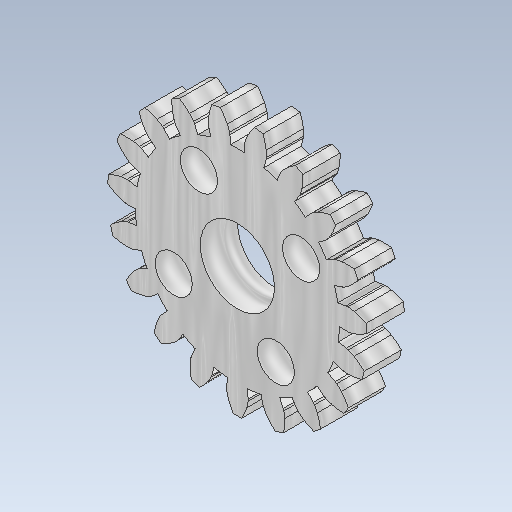
# Autodesk Inventor part: m1歯数19ギアネジ切3td5.98
Saved by Autodesk Inventor 2020.2 (Build 242310000, 310)
## iProperties
Created: 2020-02-29
Part Number: m1歯数19ギアネジ切3td5.98
Material: アルミニウム 7075
Document SubType Name: Modeling
Designer: aoyam
Density: 2.81 g/cm^3
Appearance: サテン - ブラシ仕上げ 重厚
Author: aoyam
Autodesk Inventor part; units mm, degrees
ref_plane "YZ Plane" through (0, 0, 0) normal (1, 0, 0) x (0, 1, 0)
ref_plane "XZ Plane" through (0, 0, 0) normal (0, 1, 0) x (-1, 0, 0)
ref_plane "XY Plane" through (0, 0, 0) normal (0, 0, 1) x (1, 0, 0)
sketch "スケッチ1" plane through (0, 0, 0) normal (0, 0, 1) x (1, 0, 0)
  arc A0 (2.202, 9.4851) -> (2.1723, 9.3327) centre (3.0999, 9.2311) ccw
  arc A1 (2.3854, 9.9626) -> (2.202, 9.4851) centre (4.6851, 8.8056) ccw
  arc A2 (2.953, 10.829) -> (2.3854, 9.9626) centre (6.3936, 7.9557) ccw
  arc A3 (0.9673, 9.3327) -> (0.9376, 9.4851) centre (0.0398, 9.2311) ccw
  arc A4 (0.9376, 9.4851) -> (0.7543, 9.9626) centre (-1.5454, 8.8056) ccw
  arc A5 (0.7543, 9.9626) -> (0.1867, 10.829) centre (-3.2539, 7.9557) ccw
  arc A6 (2.1266, 8.6594) -> (1.013, 8.6594) centre (1.5698, 0.4558) ccw
  arc A7 (0.1867, 10.829) -> (-0.4901, 10.716) centre (1.5698, 0.4558) ccw
  line L0 (2.1266, 8.6594) -> (2.1723, 9.3327)
  line L1 (1.013, 8.6594) -> (0.9673, 9.3327)
  line L2 (-1.6205, 8.0341) -> (-1.8823, 8.6561)
  arc A8 (-1.8823, 8.6561) -> (-1.9599, 8.7906) centre (-2.7267, 8.2588) ccw
  arc A9 (-1.9599, 8.7906) -> (-2.2884, 9.1827) centre (-4.0878, 7.3416) ccw
  arc A10 (-2.2884, 9.1827) -> (-3.1065, 9.8178) centre (-5.4278, 5.983) ccw
  arc A11 (-3.1065, 9.8178) -> (-3.71, 9.4912) centre (1.5698, 0.4558) ccw
  arc A12 (-0.764, 9.2012) -> (-0.7426, 9.0473) centre (0.1677, 9.2524) ccw
  arc A13 (-0.5672, 8.3957) -> (-1.6205, 8.0341) centre (1.5698, 0.4558) ccw
  line L3 (-0.5672, 8.3957) -> (-0.7426, 9.0473)
  arc A14 (-0.7457, 9.7123) -> (-0.764, 9.2012) centre (1.8051, 9.3647) ccw
  arc A15 (-0.4901, 10.716) -> (-0.7457, 9.7123) centre (3.697, 9.1156) ccw
  line L4 (-3.9083, 6.5876) -> (-4.3579, 7.0908)
  arc A16 (-4.3579, 7.0908) -> (-4.475, 7.1929) centre (-5.0275, 6.4409) ccw
  arc A17 (-4.475, 7.1929) -> (-4.9129, 7.4571) centre (-6.0171, 5.1315) ccw
  arc A18 (-4.9129, 7.4571) -> (-5.893, 7.7921) centre (-6.8433, 3.4114) ccw
  arc A19 (-5.893, 7.7921) -> (-6.3577, 7.2873) centre (1.5698, 0.4558) ccw
  arc A20 (-3.4772, 7.9695) -> (-3.407, 7.8309) centre (-2.6126, 8.3205) ccw
  arc A21 (-3.0295, 7.2716) -> (-3.9083, 6.5876) centre (1.5698, 0.4558) ccw
  line L5 (-3.0295, 7.2716) -> (-3.407, 7.8309)
  arc A22 (-3.6258, 8.4589) -> (-3.4772, 7.9695) centre (-1.1003, 8.9584) ccw
  arc A23 (-3.71, 9.4912) -> (-3.6258, 8.4589) centre (0.7699, 9.337) ccw
  line L6 (-5.6025, 4.4766) -> (-6.1911, 4.8066)
  arc A24 (-6.1911, 4.8066) -> (-6.335, 4.8651) centre (-6.6134, 3.9745) ccw
  arc A25 (-6.335, 4.8651) -> (-6.835, 4.9728) centre (-7.1242, 2.4147) ccw
  arc A26 (-6.835, 4.9728) -> (-7.8708, 4.9714) centre (-7.3472, 0.5195) ccw
  arc A27 (-7.8708, 4.9714) -> (-8.1464, 4.3431) centre (1.5698, 0.4558) ccw
  arc A28 (-5.6434, 5.9236) -> (-5.5321, 5.8154) centre (-4.9397, 6.5363) ccw
  arc A29 (-4.9934, 5.4089) -> (-5.6025, 4.4766) centre (1.5698, 0.4558) ccw
  line L7 (-4.9934, 5.4089) -> (-5.5321, 5.8154)
  arc A30 (-5.9429, 6.3382) -> (-5.6434, 5.9236) centre (-3.7165, 7.6307) ccw
  arc A31 (-6.3577, 7.2873) -> (-5.9429, 6.3382) centre (-2.0705, 8.5961) ccw
  line L8 (-6.5194, 1.9299) -> (-7.1833, 2.0508)
  arc A32 (-7.1833, 2.0508) -> (-7.3384, 2.0595) centre (-7.3126, 1.1267) ccw
  arc A33 (-7.3384, 2.0595) -> (-7.8463, 1.999) centre (-7.2892, -0.5144) ccw
  arc A34 (-7.8463, 1.999) -> (-8.8255, 1.6614) centre (-6.8847, -2.3793) ccw
  arc A35 (-8.8255, 1.6614) -> (-8.8821, 0.9776) centre (1.5698, 0.4558) ccw
  arc A36 (-7.028, 3.2852) -> (-6.8875, 3.219) centre (-6.5613, 4.0932) ccw
  arc A37 (-6.2461, 3.0094) -> (-6.5194, 1.9299) centre (1.5698, 0.4558) ccw
  line L9 (-6.2461, 3.0094) -> (-6.8875, 3.219)
  arc A38 (-7.4459, 3.5801) -> (-7.028, 3.2852) centre (-5.7597, 5.5255) ccw
  arc A39 (-8.1464, 4.3431) -> (-7.4459, 3.5801) centre (-4.5164, 6.973) ccw
  line L10 (-6.5598, -0.7766) -> (-7.227, -0.8777)
  arc A40 (-7.227, -0.8777) -> (-7.3765, -0.9199) centre (-7.0491, -1.7937) ccw
  arc A41 (-7.3765, -0.9199) -> (-7.8372, -1.1421) centre (-6.4942, -3.3384) ccw
  arc A42 (-7.8372, -1.1421) -> (-8.6537, -1.7793) centre (-5.5061, -4.9709) ccw
  arc A43 (-8.6537, -1.7793) -> (-8.4853, -2.4444) centre (1.5698, 0.4558) ccw
  arc A44 (-7.4809, 0.3402) -> (-7.3265, 0.3232) centre (-7.3019, 1.2559) ccw
  arc A45 (-6.6517, 0.3332) -> (-6.5598, -0.7766) centre (1.5698, 0.4558) ccw
  line L11 (-6.6517, 0.3332) -> (-7.3265, 0.3232)
  arc A46 (-7.9719, 0.4835) -> (-7.4809, 0.3402) centre (-7.0087, 2.8709) ccw
  arc A47 (-8.8821, 0.9776) -> (-7.9719, 0.4835) centre (-6.3028, 4.6437) ccw
  line L12 (-5.7192, -3.3495) -> (-6.3174, -3.6618)
  arc A48 (-6.3174, -3.6618) -> (-6.445, -3.7502) centre (-5.8517, -4.4704) ccw
  arc A49 (-6.445, -3.7502) -> (-6.8087, -4.1099) centre (-4.8253, -5.7512) ccw
  arc A50 (-6.8087, -4.1099) -> (-7.374, -4.9778) centre (-3.3607, -6.9744) ccw
  arc A51 (-7.374, -4.9778) -> (-6.9988, -5.5522) centre (1.5698, 0.4558) ccw
  arc A52 (-6.953, -2.5923) -> (-6.8014, -2.5583) centre (-7.081, -1.6681) ccw
  arc A53 (-6.1665, -2.3297) -> (-5.7192, -3.3495) centre (1.5698, 0.4558) ccw
  line L13 (-6.1665, -2.3297) -> (-6.8014, -2.5583)
  arc A54 (-7.4639, -2.6162) -> (-6.953, -2.5923) centre (-7.3281, -0.0455) ccw
  arc A55 (-8.4853, -2.4444) -> (-7.4639, -2.6162) centre (-7.236, 1.8605) ccw
  line L14 (-4.0886, -5.5101) -> (-4.553, -5.9997)
  arc A56 (-4.553, -5.9997) -> (-4.6451, -6.1248) centre (-3.8501, -6.6133) ccw
  arc A57 (-4.6451, -6.1248) -> (-4.8722, -6.5831) centre (-2.4634, -7.4914) ccw
  arc A58 (-4.8722, -6.5831) -> (-5.1252, -7.5874) centre (-0.681, -8.1727) ccw
  arc A59 (-5.1252, -7.5874) -> (-4.5837, -8.0089) centre (1.5698, 0.4558) ccw
  arc A60 (-5.5015, -5.1945) -> (-5.3692, -5.1131) centre (-5.9227, -4.3619) ccw
  arc A61 (-4.8429, -4.6907) -> (-4.0886, -5.5101) centre (1.5698, 0.4558) ccw
  line L15 (-4.8429, -4.6907) -> (-5.3692, -5.1131)
  arc A62 (-5.9769, -5.383) -> (-5.5015, -5.1945) centre (-6.6832, -2.9075) ccw
  arc A63 (-6.9988, -5.5522) -> (-5.9769, -5.383) centre (-7.2151, -1.0748) ccw
  line L16 (-1.845, -7.0241) -> (-2.1252, -7.638)
  arc A64 (-2.1252, -7.638) -> (-2.1717, -7.7862) centre (-1.2611, -7.9901) ccw
  arc A65 (-2.1717, -7.7862) -> (-2.2377, -8.2934) centre (0.3356, -8.3704) ccw
  arc A66 (-2.2377, -8.2934) -> (-2.1508, -9.3255) centre (2.2426, -8.4361) ccw
  arc A67 (-2.1508, -9.3255) -> (-1.5018, -9.5483) centre (1.5698, 0.4558) ccw
  arc A68 (-3.2837, -7.1844) -> (-3.185, -7.0645) centre (-3.9524, -6.5337) ccw
  arc A69 (-2.8243, -6.4941) -> (-1.845, -7.0241) centre (1.5698, 0.4558) ccw
  line L17 (-2.8243, -6.4941) -> (-3.185, -7.0645)
  arc A70 (-3.6722, -7.5171) -> (-3.2837, -7.1844) centre (-5.144, -5.405) ccw
  arc A71 (-4.5837, -8.0089) -> (-3.6722, -7.5171) centre (-6.2421, -3.8444) ccw
  line L18 (0.7688, -7.7276) -> (0.703, -8.3992)
  arc A72 (0.703, -8.3992) -> (0.7072, -8.5545) centre (1.6347, -8.4517) ccw
  arc A73 (0.7072, -8.5545) -> (0.8095, -9.0556) centre (3.2683, -8.2929) ccw
  arc A74 (0.8095, -9.0556) -> (1.2268, -10.0036) centre (5.0934, -7.7358) ccw
  arc A75 (1.2268, -10.0036) -> (1.9129, -10.0036) centre (1.5698, 0.4558) ccw
  arc A76 (-0.5399, -8.3464) -> (-0.4855, -8.2009) centre (-1.3837, -7.948) ccw
  arc A77 (-0.3296, -7.5443) -> (0.7688, -7.7276) centre (1.5698, 0.4558) ccw
  line L19 (-0.3296, -7.5443) -> (-0.4855, -8.2009)
  arc A78 (-0.7994, -8.7872) -> (-0.5399, -8.3464) centre (-2.8773, -7.2674) ccw
  arc A79 (-1.5018, -9.5483) -> (-0.7994, -8.7872) centre (-4.4226, -6.1479) ccw
  line L20 (3.4693, -7.5443) -> (3.6252, -8.2009)
  arc A80 (3.6252, -8.2009) -> (3.6796, -8.3464) centre (4.5234, -7.948) ccw
  arc A81 (3.6796, -8.3464) -> (3.939, -8.7872) centre (6.0169, -7.2674) ccw
  arc A82 (3.939, -8.7872) -> (4.6415, -9.5483) centre (7.5622, -6.1479) ccw
  arc A83 (4.6415, -9.5483) -> (5.2905, -9.3255) centre (1.5698, 0.4558) ccw
  arc A84 (2.4324, -8.5545) -> (2.4366, -8.3992) centre (1.505, -8.4517) ccw
  arc A85 (2.3709, -7.7276) -> (3.4693, -7.5443) centre (1.5698, 0.4558) ccw
  line L21 (2.3709, -7.7276) -> (2.4366, -8.3992)
  arc A86 (2.3302, -9.0556) -> (2.4324, -8.5545) centre (-0.1286, -8.2929) ccw
  arc A87 (1.9129, -10.0036) -> (2.3302, -9.0556) centre (-1.9537, -7.7358) ccw
  line L22 (5.964, -6.4941) -> (6.3247, -7.0645)
  arc A88 (6.3247, -7.0645) -> (6.4233, -7.1844) centre (7.0921, -6.5337) ccw
  arc A89 (6.4233, -7.1844) -> (6.8118, -7.5171) centre (8.2837, -5.405) ccw
  arc A90 (6.8118, -7.5171) -> (7.7234, -8.0089) centre (9.3818, -3.8444) ccw
  arc A91 (7.7234, -8.0089) -> (8.2649, -7.5874) centre (1.5698, 0.4558) ccw
  arc A92 (5.3113, -7.7862) -> (5.2649, -7.638) centre (4.4008, -7.9901) ccw
  arc A93 (4.9846, -7.0241) -> (5.964, -6.4941) centre (1.5698, 0.4558) ccw
  line L23 (4.9846, -7.0241) -> (5.2649, -7.638)
  arc A94 (5.3773, -8.2934) -> (5.3113, -7.7862) centre (2.8041, -8.3704) ccw
  arc A95 (5.2905, -9.3255) -> (5.3773, -8.2934) centre (0.897, -8.4361) ccw
  line L24 (7.9826, -4.6907) -> (8.5089, -5.1131)
  arc A96 (8.5089, -5.1131) -> (8.6411, -5.1945) centre (9.0623, -4.3619) ccw
  arc A97 (8.6411, -5.1945) -> (9.1166, -5.383) centre (9.8229, -2.9075) ccw
  arc A98 (9.1166, -5.383) -> (10.1384, -5.5522) centre (10.3547, -1.0748) ccw
  arc A99 (10.1384, -5.5522) -> (10.5137, -4.9778) centre (1.5698, 0.4558) ccw
  arc A100 (7.7848, -6.1248) -> (7.6927, -5.9997) centre (6.9898, -6.6133) ccw
  arc A101 (7.2283, -5.5101) -> (7.9826, -4.6907) centre (1.5698, 0.4558) ccw
  line L25 (7.2283, -5.5101) -> (7.6927, -5.9997)
  arc A102 (8.0119, -6.5831) -> (7.7848, -6.1248) centre (5.6031, -7.4914) ccw
  arc A103 (8.2649, -7.5874) -> (8.0119, -6.5831) centre (3.8207, -8.1727) ccw
  line L26 (9.3062, -2.3297) -> (9.9411, -2.5583)
  arc A104 (9.9411, -2.5583) -> (10.0926, -2.5923) centre (10.2207, -1.6681) ccw
  arc A105 (10.0926, -2.5923) -> (10.6035, -2.6162) centre (10.4678, -0.0455) ccw
  arc A106 (10.6035, -2.6162) -> (11.6249, -2.4444) centre (10.3757, 1.8605) ccw
  arc A107 (11.6249, -2.4444) -> (11.7934, -1.7793) centre (1.5698, 0.4558) ccw
  arc A108 (9.5847, -3.7502) -> (9.457, -3.6618) centre (8.9914, -4.4704) ccw
  arc A109 (8.8588, -3.3495) -> (9.3062, -2.3297) centre (1.5698, 0.4558) ccw
  line L27 (8.8588, -3.3495) -> (9.457, -3.6618)
  arc A110 (9.9483, -4.1099) -> (9.5847, -3.7502) centre (7.965, -5.7512) ccw
  arc A111 (10.5137, -4.9778) -> (9.9483, -4.1099) centre (6.5004, -6.9744) ccw
  line L28 (9.7914, 0.3332) -> (10.4662, 0.3232)
  arc A112 (10.4662, 0.3232) -> (10.6206, 0.3402) centre (10.4415, 1.2559) ccw
  arc A113 (10.6206, 0.3402) -> (11.1115, 0.4835) centre (10.1484, 2.8709) ccw
  arc A114 (11.1115, 0.4835) -> (12.0218, 0.9776) centre (9.4425, 4.6437) ccw
  arc A115 (12.0218, 0.9776) -> (11.9652, 1.6614) centre (1.5698, 0.4558) ccw
  arc A116 (10.5162, -0.9199) -> (10.3667, -0.8777) centre (10.1888, -1.7937) ccw
  arc A117 (9.6995, -0.7766) -> (9.7914, 0.3332) centre (1.5698, 0.4558) ccw
  line L29 (9.6995, -0.7766) -> (10.3667, -0.8777)
  arc A118 (10.9768, -1.1421) -> (10.5162, -0.9199) centre (9.6339, -3.3384) ccw
  arc A119 (11.7934, -1.7793) -> (10.9768, -1.1421) centre (8.6458, -4.9709) ccw
  line L30 (9.3858, 3.0094) -> (10.0272, 3.219)
  arc A120 (10.0272, 3.219) -> (10.1677, 3.2852) centre (9.701, 4.0932) ccw
  arc A121 (10.1677, 3.2852) -> (10.5856, 3.5801) centre (8.8994, 5.5255) ccw
  arc A122 (10.5856, 3.5801) -> (11.2861, 4.3431) centre (7.6561, 6.973) ccw
  arc A123 (11.2861, 4.3431) -> (11.0104, 4.9714) centre (1.5698, 0.4558) ccw
  arc A124 (10.4781, 2.0595) -> (10.323, 2.0508) centre (10.4522, 1.1267) ccw
  arc A125 (9.6591, 1.9299) -> (9.3858, 3.0094) centre (1.5698, 0.4558) ccw
  line L31 (9.6591, 1.9299) -> (10.323, 2.0508)
  arc A126 (10.986, 1.999) -> (10.4781, 2.0595) centre (10.4289, -0.5144) ccw
  arc A127 (11.9652, 1.6614) -> (10.986, 1.999) centre (10.0244, -2.3793) ccw
  line L32 (8.1331, 5.4089) -> (8.6717, 5.8154)
  arc A128 (8.6717, 5.8154) -> (8.7831, 5.9236) centre (8.0794, 6.5363) ccw
  arc A129 (8.7831, 5.9236) -> (9.0826, 6.3382) centre (6.8562, 7.6307) ccw
  arc A130 (9.0826, 6.3382) -> (9.4974, 7.2873) centre (5.2102, 8.5961) ccw
  arc A131 (9.4974, 7.2873) -> (9.0327, 7.7921) centre (1.5698, 0.4558) ccw
  arc A132 (9.4747, 4.8651) -> (9.3308, 4.8066) centre (9.7531, 3.9745) ccw
  arc A133 (8.7422, 4.4766) -> (8.1331, 5.4089) centre (1.5698, 0.4558) ccw
  line L33 (8.7422, 4.4766) -> (9.3308, 4.8066)
  arc A134 (9.9747, 4.9728) -> (9.4747, 4.8651) centre (10.2639, 2.4147) ccw
  arc A135 (11.0104, 4.9714) -> (9.9747, 4.9728) centre (10.4869, 0.5195) ccw
  line L34 (6.1692, 7.2716) -> (6.5467, 7.8309)
  arc A136 (6.5467, 7.8309) -> (6.6169, 7.9695) centre (5.7523, 8.3205) ccw
  arc A137 (6.6169, 7.9695) -> (6.7655, 8.4589) centre (4.24, 8.9584) ccw
  arc A138 (6.7655, 8.4589) -> (6.8497, 9.4912) centre (2.3698, 9.337) ccw
  arc A139 (6.8497, 9.4912) -> (6.2462, 9.8178) centre (1.5698, 0.4558) ccw
  arc A140 (7.6147, 7.1929) -> (7.4976, 7.0908) centre (8.1672, 6.4409) ccw
  arc A141 (7.048, 6.5876) -> (6.1692, 7.2716) centre (1.5698, 0.4558) ccw
  line L35 (7.048, 6.5876) -> (7.4976, 7.0908)
  arc A142 (8.0526, 7.4571) -> (7.6147, 7.1929) centre (9.1568, 5.1315) ccw
  arc A143 (9.0327, 7.7921) -> (8.0526, 7.4571) centre (9.983, 3.4114) ccw
  line L36 (3.7069, 8.3957) -> (3.8823, 9.0473)
  arc A144 (3.8823, 9.0473) -> (3.9037, 9.2012) centre (2.972, 9.2524) ccw
  arc A145 (3.9037, 9.2012) -> (3.8853, 9.7123) centre (1.3346, 9.3647) ccw
  arc A146 (3.8853, 9.7123) -> (3.6298, 10.716) centre (-0.5573, 9.1156) ccw
  arc A147 (3.6298, 10.716) -> (2.953, 10.829) centre (1.5698, 0.4558) ccw
  arc A148 (5.0996, 8.7906) -> (5.022, 8.6561) centre (5.8663, 8.2588) ccw
  arc A149 (4.7602, 8.0341) -> (3.7069, 8.3957) centre (1.5698, 0.4558) ccw
  line L37 (4.7602, 8.0341) -> (5.022, 8.6561)
  arc A150 (5.4281, 9.1827) -> (5.0996, 8.7906) centre (7.2275, 7.3416) ccw
  arc A151 (6.2462, 9.8178) -> (5.4281, 9.1827) centre (8.5674, 5.983) ccw
  circle A152 centre (1.5698, 0.4558) radius 2.99
  circle A153 centre (-1.531, 5.5924) radius 1.495
  circle A154 centre (-3.5668, -2.645) radius 1.495
  circle A155 centre (4.6706, -4.6809) radius 1.495
  circle A156 centre (6.7065, 3.5566) radius 1.495
  point P0 (0, 0)
  point P1 (-5.6025, 4.4766)
  point P2 (-6.1911, 4.8066)
  point P3 (-6.335, 4.8651)
  point P4 (-6.835, 4.9728)
  point P5 (-7.8708, 4.9714)
  point P6 (-8.1464, 4.3431)
  point P7 (-7.4459, 3.5801)
  point P8 (-7.028, 3.2852)
  point P9 (-6.8875, 3.219)
  point P10 (-6.2461, 3.0094)
  point P11 (-6.5194, 1.9299)
  point P12 (-7.1833, 2.0508)
  point P13 (-7.3384, 2.0595)
  point P14 (-7.8463, 1.999)
  point P15 (-8.8255, 1.6614)
  point P16 (-8.8821, 0.9776)
  point P17 (-7.9719, 0.4835)
  point P18 (-7.4809, 0.3402)
  point P19 (-7.227, -0.8777)
  point P20 (-7.3765, -0.9199)
  point P21 (-7.8372, -1.1421)
  point P22 (-8.6537, -1.7793)
  point P23 (-8.4853, -2.4444)
  point P24 (-7.4639, -2.6162)
  point P25 (-6.953, -2.5923)
  point P26 (-6.8014, -2.5583)
  point P27 (-6.445, -3.7502)
  point P28 (-6.8087, -4.1099)
  point P29 (-7.374, -4.9778)
  point P30 (-6.9988, -5.5522)
  point P31 (-5.9769, -5.383)
  point P32 (-5.5015, -5.1945)
  point P33 (-4.6451, -6.1248)
  point P34 (-4.8722, -6.5831)
  point P35 (-5.1252, -7.5874)
  point P36 (-4.5837, -8.0089)
  point P37 (-3.6722, -7.5171)
  point P38 (-3.2837, -7.1844)
  point P39 (-2.1717, -7.7862)
  point P40 (-2.2377, -8.2934)
  point P41 (-2.1508, -9.3255)
  point P42 (-1.5018, -9.5483)
  point P43 (-0.7994, -8.7872)
  point P44 (-0.5399, -8.3464)
  point P45 (-0.4855, -8.2009)
  point P46 (0.7072, -8.5545)
  point P47 (0.8095, -9.0556)
  point P48 (1.2268, -10.0036)
  point P49 (1.9129, -10.0036)
  point P50 (2.3302, -9.0556)
  point P51 (2.4324, -8.5545)
  point P52 (2.3709, -7.7276)
  point P53 (3.6796, -8.3464)
  point P54 (3.939, -8.7872)
  point P55 (4.6415, -9.5483)
  point P56 (5.2905, -9.3255)
  point P57 (5.3773, -8.2934)
  point P58 (5.3113, -7.7862)
  point P59 (5.2649, -7.638)
  point P60 (4.9846, -7.0241)
  point P61 (5.964, -6.4941)
  point P62 (6.4233, -7.1844)
  point P63 (6.8118, -7.5171)
  point P64 (7.7234, -8.0089)
  point P65 (8.2649, -7.5874)
  point P66 (8.0119, -6.5831)
  point P67 (7.7848, -6.1248)
  point P68 (7.6927, -5.9997)
  point P69 (7.2283, -5.5101)
  point P70 (8.5089, -5.1131)
  point P71 (8.6411, -5.1945)
  point P72 (9.1166, -5.383)
  point P73 (10.1384, -5.5522)
  point P74 (10.5137, -4.9778)
  point P75 (9.9483, -4.1099)
  point P76 (9.5847, -3.7502)
  point P77 (9.457, -3.6618)
  point P78 (8.8588, -3.3495)
  point P79 (9.3062, -2.3297)
  point P80 (9.9411, -2.5583)
  point P81 (10.0926, -2.5923)
  point P82 (10.6035, -2.6162)
  point P83 (11.6249, -2.4444)
  point P84 (11.7934, -1.7793)
  point P85 (10.9768, -1.1421)
  point P86 (10.5162, -0.9199)
  point P87 (10.3667, -0.8777)
  point P88 (9.6995, -0.7766)
  point P89 (9.7914, 0.3332)
  point P90 (10.4662, 0.3232)
  point P91 (10.6206, 0.3402)
  point P92 (11.1115, 0.4835)
  point P93 (12.0218, 0.9776)
  point P94 (11.9652, 1.6614)
  point P95 (10.986, 1.999)
  point P96 (10.4781, 2.0595)
  point P97 (9.6591, 1.9299)
  point P98 (10.1677, 3.2852)
  point P99 (10.5856, 3.5801)
  point P100 (11.2861, 4.3431)
  point P101 (11.0104, 4.9714)
  point P102 (9.9747, 4.9728)
  point P103 (9.4747, 4.8651)
  point P104 (9.3308, 4.8066)
  point P105 (8.7422, 4.4766)
  point P106 (8.1331, 5.4089)
  point P107 (8.6717, 5.8154)
  point P108 (8.7831, 5.9236)
  point P109 (9.0826, 6.3382)
  point P110 (9.4974, 7.2873)
  point P111 (9.0327, 7.7921)
  point P112 (8.0526, 7.4571)
  point P113 (7.6147, 7.1929)
  point P114 (7.048, 6.5876)
  point P115 (6.1692, 7.2716)
  point P116 (6.5467, 7.8309)
  point P117 (6.6169, 7.9695)
  point P118 (6.7655, 8.4589)
  point P119 (6.8497, 9.4912)
  point P120 (6.2462, 9.8178)
  point P121 (5.4281, 9.1827)
  point P122 (5.0996, 8.7906)
  point P123 (5.022, 8.6561)
  point P124 (4.7602, 8.0341)
  point P125 (3.9037, 9.2012)
  point P126 (3.8853, 9.7123)
  point P127 (3.6298, 10.716)
  point P128 (2.953, 10.829)
  point P129 (2.3854, 9.9626)
  point P130 (2.202, 9.4851)
  point P131 (0.9376, 9.4851)
  point P132 (0.7543, 9.9626)
  point P133 (0.1867, 10.829)
  point P134 (-0.4901, 10.716)
  point P135 (-0.7457, 9.7123)
  point P136 (-0.764, 9.2012)
  point P137 (-0.7426, 9.0473)
  point P138 (-1.8823, 8.6561)
  point P139 (-1.9599, 8.7906)
  point P140 (-2.2884, 9.1827)
  point P141 (-3.1065, 9.8178)
  point P142 (-3.71, 9.4912)
  point P143 (-3.6258, 8.4589)
  point P144 (-3.4772, 7.9695)
  point P145 (-3.407, 7.8309)
  point P146 (-3.0295, 7.2716)
  point P147 (-3.9083, 6.5876)
  point P148 (-4.3579, 7.0908)
  point P149 (-4.475, 7.1929)
  point P150 (-4.9129, 7.4571)
  point P151 (-5.893, 7.7921)
  point P152 (-6.3577, 7.2873)
  point P153 (-5.9429, 6.3382)
  point P154 (-5.6434, 5.9236)
  dimension "d2" = 360
  dimension "d4" = 5.98
  dimension "d5" = 2.99
  dimension "d6" = 6
  dimension "d9" = 360
  constraints: 304 point on circle, 157 centre point, 76 end point, 2 coincident, 730 other
  measures "d4" diameter of A152
  measures "d5" diameter of A153
  measures "d6" distance of A153.centre A6.centre
extrude "押し出し1" add sketch "スケッチ1" along normal blind 3
